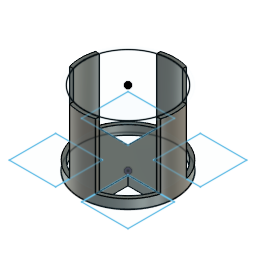
アトマイザー固定治具3 (Autodesk Fusion 360 design; units mm, degrees)
Autodesk Fusion 360 part; units mm, degrees
sketch "スケッチ1" plane through (0, 0, 0) normal (0, 0, 1) x (1, 0, 0)
  circle A0 centre (0, 0) radius 25.5
  dimension "d1" = 51
  constraint coincident A0.centre origin
  measures "d1" diameter of A0
extrude "押し出し1" add sketch "スケッチ1" along normal blind 40
sketch "スケッチ2" plane through (0, 0, 40) normal (0, 0, 1) x (-1, 0, 0)
  circle A0 centre (0, 0) radius 25.5
  circle A1 centre (0, 0) radius 23.5
  dimension "d4" = 47
  constraint coincident A0.centre A1.centre
  measures "d4" diameter of A1
extrude "押し出し2" cut sketch "スケッチ2" against normal blind 35 contours A1
sketch "スケッチ3" plane through (0, 0, 5) normal (0, 0, 1) x (-1, 0, 0)
  circle A0 centre (0, 0) radius 23.5
  line L0 (7, -7) -> (32, -7)
  line L1 (32, -7) -> (32, -32)
  line L2 (32, -32) -> (7, -32)
  line L3 (7, -32) -> (7, -7)
  line L4 (7, 7) -> (32, 7)
  line L5 (32, 7) -> (32, 32)
  line L6 (32, 32) -> (7, 32)
  line L7 (7, 32) -> (7, 7)
  line L8 (-7, 7) -> (-32, 7)
  line L9 (-32, 7) -> (-32, 32)
  line L10 (-32, 32) -> (-7, 32)
  line L11 (-7, 32) -> (-7, 7)
  line L12 (-7, -7) -> (-32, -7)
  line L13 (-32, -7) -> (-32, -32)
  line L14 (-32, -32) -> (-7, -32)
  line L15 (-7, -32) -> (-7, -7)
  dimension "d7" = 25
  dimension "d8" = 25
  dimension "d9" = 25
  dimension "d10" = 25
  dimension "d11" = 25
  dimension "d12" = 25
  dimension "d13" = 25
  dimension "d14" = 25
  constraint horizontal L0
  constraint vertical L1
  constraint horizontal L2
  constraint vertical L3
  constraint horizontal L4
  constraint vertical L5
  constraint horizontal L6
  constraint vertical L7
  constraint horizontal L8
  constraint vertical L9
  constraint horizontal L10
  constraint vertical L11
  constraint horizontal L12
  constraint vertical L13
  constraint horizontal L14
  constraint vertical L15
  measures "d7" distance of L0.end L1.end
  measures "d8" distance of L1.end L2.end
  measures "d9" distance of L5.end L6.end
  measures "d10" distance of L4.end L5.end
  measures "d11" distance of L9.end L10.end
  measures "d12" distance of L8.end L9.end
  measures "d13" distance of L12.end L13.end
  measures "d14" distance of L13.end L14.end
extrude "押し出し3" cut sketch "スケッチ3" along normal blind 35 contours A0 L12 L13 L14 L15
extrude "押し出し4" cut sketch "スケッチ3" along normal blind 35 contours A0 L0 L1 L2 L3
extrude "押し出し5" cut sketch "スケッチ3" along normal blind 35 contours A0 L4 L5 L6 L7 | A0 L8 L9 L10 L11
extrude "押し出し6" cut sketch "スケッチ3" against normal blind 5 contours A0 L4 L7 | A0 L0 L3 | A0 L8 L11 | A0 L12 L15
